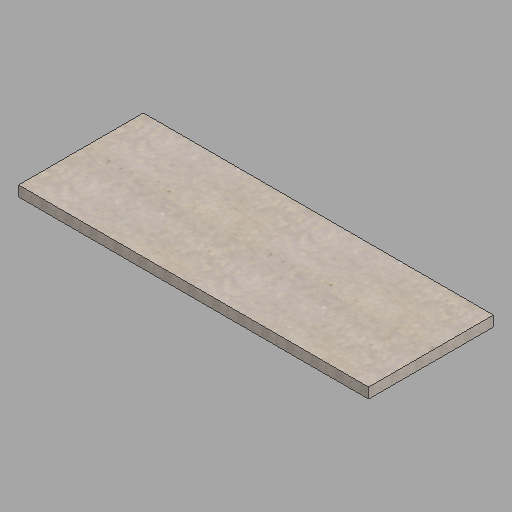
# Autodesk Inventor part: StoneLid
Saved by Autodesk Inventor 2022.1 (Build 261234020, 234B)
## iProperties
Created: 2021-10-22
Part Number: StoneLid
Material: Limestone
Document SubType Name: Modeling
Designer: awelt
Density: 2.6 g/cm^3
Appearance: Kasota Gray
Mass: 464750 g
Surface Area: 52219.3 cm^2
Volume: 178750 cm^3
Author: awelt
Autodesk Inventor part; units mm, degrees
ref_plane "YZ Plane" through (0, 0, 0) normal (1, 0, 0) x (0, 1, 0)
ref_plane "XZ Plane" through (0, 0, 0) normal (0, 1, 0) x (-1, 0, 0)
ref_plane "XY Plane" through (0, 0, 0) normal (0, 0, 1) x (1, 0, 0)
sketch "Sketch1" plane through (0, 0, 0) normal (0, 1, 0) x (-1, 0, 0)
  line L0 (1282.7, -457.2) -> (-1282.7, -457.2)
  line L1 (-1282.7, -457.2) -> (-1282.7, 457.2)
  line L2 (-1282.7, 457.2) -> (1282.7, 457.2)
  line L3 (1282.7, 457.2) -> (1282.7, -457.2)
  line L4 (1282.7, -457.2) -> (-1282.7, 457.2) construction
  line L5 (-1282.7, -457.2) -> (1282.7, 457.2) construction
  point P0 (0, 0)
  dimension "d0" = 2565.4
  dimension "d1" = 914.4
  constraints: 12 end point, 2 midpoint, 2 parallel, 1 horizontal, 1 perpendicular
  measures "d0" distance of L1.end L2.end
  measures "d1" distance of L0.end L1.end
extrude "Extrusion1" add sketch "Sketch1" along normal blind 76.2
